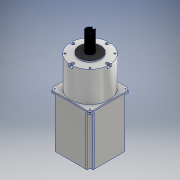
# Autodesk Inventor part: Nema 23 Stepper Motor
Saved by Autodesk Inventor 2018 (Build 220112000, 112)
## iProperties
Created: 2017-11-21
Part Number: Nema 23 Stepper Motor
Material: Generic
Document SubType Name: Modeling
Designer: p447144
Density: 1 g/cm^3
Appearance: Aluminum - Flat
Author: p447144
Autodesk Inventor part; units mm, degrees
ref_plane "YZ Plane" through (0, 0, 0) normal (1, 0, 0) x (0, 1, 0)
ref_plane "XY Plane" through (0, 0, 0) normal (0, 0, 1) x (1, 0, 0)
sketch "Sketch1" plane through (0, 0, 0) normal (0, 0, 1) x (1, 0, 0)
  line L0 (-28.5, -28.5) -> (28.5, -28.5)
  line L1 (28.5, -28.5) -> (28.5, 28.5)
  line L2 (28.5, 28.5) -> (-28.5, 28.5)
  line L3 (-28.5, 28.5) -> (-28.5, -28.5)
  arc A0 (23.5, 28.5) -> (28.5, 23.5) centre (28.5, 28.5) ccw
  line L4 (0, 28.5) -> (0, -28.5) construction
  line L5 (-28.5, 0) -> (28.5, 0) construction
  arc A1 (-28.5, 23.5) -> (-23.5, 28.5) centre (-28.5, 28.5) ccw
  arc A2 (28.5, -23.5) -> (23.5, -28.5) centre (28.5, -28.5) ccw
  arc A3 (-23.5, -28.5) -> (-28.5, -23.5) centre (-28.5, -28.5) ccw
  point P0 (0, 0)
  dimension "d0" = 57
  dimension "d1" = 57
  dimension "d2" = 10
  constraints: 12 end point, 8 point on circle, 8 point on line, 4 centre point, 4 midpoint, 3 symmetric about line, 2 parallel, 1 coincident, 1 horizontal, 1 perpendicular, 3 other
  measures "d0" distance of L2.end L1.end
  measures "d1" distance of L1.end L0.end
  measures "d2" diameter of A0
extrude "Extrusion1" add sketch "Sketch1" along normal blind 73 contours A3 L3 A1 L2 A0 L1 A2 L0
sketch "Sketch2" plane through (0, 0, 73) normal (0, 0, 1) x (1, 0, 0)
  line L0 (-28.5, -28.5) -> (28.5, -28.5)
  line L1 (28.5, -28.5) -> (28.5, 28.5)
  line L2 (28.5, 28.5) -> (-28.5, 28.5)
  line L3 (-28.5, 28.5) -> (-28.5, -28.5)
  line L4 (-28.5, -28.5) -> (28.5, 28.5) construction
  line L5 (28.5, -28.5) -> (-28.5, 28.5) construction
  point P0 (0, 0)
  dimension "d5" = 57
  dimension "d6" = 57
  constraints: 12 end point, 2 midpoint, 2 parallel, 1 horizontal, 1 perpendicular
  measures "d5" distance of L2.end L1.end
  measures "d6" distance of L1.end L0.end
extrude "Extrusion2" add sketch "Sketch2" along normal blind 3
sketch "Sketch3" plane through (0, 0, 76) normal (0, 0, 1) x (1, 0, 0)
  arc A0 (-28.5, 23.5) -> (-23.5, 28.5) centre (-28.5, 28.5) ccw projected
  line L0 (-28.5, 23.5) -> (-18.5, 23.5) construction
  line L1 (-23.5, 28.5) -> (-28.5, 28.5) projected
  line L2 (-23.5, 28.5) -> (-23.5, 18.5) construction
  line L3 (-23.5, 28.5) -> (-13.5, 28.5) construction
  line L4 (-28.5, 28.5) -> (-23.5, 23.5) construction
  line L5 (-23.5, 28.5) -> (-28.5, 23.5) construction
  circle A1 centre (-26, 26) radius 0.75
  line L6 (23.5, 28.5) -> (-23.5, 28.5) projected
  line L7 (0, 28.5) -> (0, -28.5) construction
  line L8 (-23.5, -28.5) -> (23.5, -28.5) projected
  line L9 (28.5, -23.5) -> (28.5, 23.5) projected
  line L10 (-28.5, 23.5) -> (-28.5, -23.5) projected
  line L11 (-28.5, 0) -> (28.5, 0) construction
  circle A2 centre (26, 26) radius 0.75
  line L12 (28.5, 0) -> (-28.5, 0) construction
  circle A3 centre (-26, -26) radius 0.75
  circle A4 centre (26, -26) radius 0.75
  point P0 (0, 0)
  dimension "d9" = 10
  dimension "d11" = 10
  dimension "d12" = 90
  dimension "d13" = 1.5
  constraints: 16 end point, 6 midpoint, 5 symmetric about line, 4 centre point, 2 horizontal, 1 perpendicular, 1 tangent, 1 vertical, 3 other
  measures "d9" distance of L0.start L0.end
  measures "d11" distance of L1.start L2.end
  measures "d12" angle of L2 L3
  measures "d13" diameter of A1
extrude "Extrusion3" cut sketch "Sketch3" against normal blind 3
sketch "Sketch4" plane through (0, 0, 76) normal (0, 0, 1) x (1, 0, 0)
  line L0 (-29.5, -29.5) -> (29.5, -29.5)
  line L1 (29.5, -29.5) -> (29.5, 29.5)
  line L2 (29.5, 29.5) -> (-29.5, 29.5)
  line L3 (-29.5, 29.5) -> (-29.5, -29.5)
  line L4 (29.5, -29.5) -> (-29.5, 29.5) construction
  line L5 (-29.5, 26) -> (-26, 29.5)
  line L6 (0, 29.5) -> (0, -29.5) construction
  line L7 (-29.5, 0) -> (29.5, 0) construction
  line L8 (29.5, 26) -> (26, 29.5)
  line L9 (-26, -29.5) -> (-29.5, -26)
  line L10 (26, -29.5) -> (29.5, -26)
  point P0 (0, 0)
  dimension "d16" = 59
  dimension "d17" = 59
  constraints: 22 end point, 8 point on line, 5 midpoint, 2 parallel, 2 perpendicular, 1 horizontal
  measures "d16" distance of L2.end L1.end
  measures "d17" distance of L1.end L0.end
extrude "Extrusion4" add sketch "Sketch4" along normal blind 2 contours L9 L3 L5 L2 L8 L1 L10 L0
sketch "Sketch5" plane through (0, 0, 78) normal (0, 0, 1) x (1, 0, 0)
  circle A0 centre (26, 26) radius 0.75 projected
  circle A1 centre (26, -26) radius 0.75 projected
  circle A2 centre (-26, -26) radius 0.75 projected
  circle A3 centre (-26, 26) radius 0.75 projected
  circle A4 centre (-26, 26) radius 0.75 projected
  circle A5 centre (-26, 26) radius 0.75
  circle A6 centre (26, 26) radius 0.75
  circle A7 centre (26, -26) radius 0.75
  circle A8 centre (-26, -26) radius 0.75
  point P0 (0, 0)
  constraints: 4 centre point, 4 coincident, 3 concentric
extrude "Extrusion5" cut sketch "Sketch5" against normal blind 2
sketch "Sketch6" plane through (0, 0, 78) normal (0, 0, 1) x (1, 0, 0)
  circle A0 centre (0, 0) radius 28.5
  constraints: 1 centre point, 1 coincident
extrude "Extrusion6" add sketch "Sketch6" along normal blind 45
sketch "Sketch7" plane through (0, 0, 123) normal (0, 0, 1) x (1, 0, 0)
  circle A0 centre (0, 0) radius 22.5 construction
  circle A1 centre (0, 0) radius 25 construction
  arc A2 (2, -25) -> (-2, -25) centre (0, -25) ccw
  circle A3 centre (0, 0) radius 28.5 projected
  line L0 (28.5, -27) -> (28.5, 27) projected
  line L1 (-28.5, 27) -> (-28.5, -27) projected
  line L2 (-23.5, -28.5) -> (23.5, -28.5) projected
  line L3 (-2, -23.5) -> (4, -23.5) construction
  line L4 (-2, -24.9199) -> (-2, -28.4297)
  line L5 (2, -24.9199) -> (2, -28.4297)
  arc A4 (-25, -2) -> (-25, 2) centre (-25, 0) ccw
  line L6 (-29.5, 26) -> (-29.5, -26) projected
  line L7 (-23, 2) -> (-15, 2) construction
  line L8 (-24.9199, 2) -> (-28.4297, 2)
  line L9 (-24.9199, -2) -> (-28.4297, -2)
  arc A5 (-2, 25) -> (2, 25) centre (0, 25) ccw
  line L10 (-2, 20.4297) -> (-2, 28.4297)
  line L11 (2, 20.4297) -> (2, 28.4297)
  line L12 (2, 20.4297) -> (10, 20.4297) construction
  line L13 (29.5, -26) -> (29.5, 26) projected
  arc A6 (25.08, 1.9984) -> (25.08, -1.9984) centre (25, 0) ccw
  line L14 (24.92, -1.9984) -> (28.4299, -1.9984)
  line L15 (24.92, 1.9984) -> (28.4299, 1.9984)
  circle A7 centre (-15, 16.7705) radius 1.5
  circle A8 centre (15, 16.7705) radius 1.5
  circle A9 centre (15, -16.7705) radius 1.5
  circle A10 centre (-15, -16.7705) radius 1.5
  circle A11 centre (-15, 16.7705) radius 1.5
  dimension "d26" = 50
  dimension "d25" = 45
  dimension "d28" = 4
  dimension "d32" = 4
  dimension "d39" = 4
  dimension "d40" = 8
  dimension "d41" = 8
  dimension "d42" = 90
  dimension "d46" = 4
  dimension "d83" = 3
  dimension "d84" = 3
  dimension "d85" = 3
  dimension "d86" = 3
  constraints: 22 end point, 14 point on circle, 10 centre point, 8 point on line, 5 horizontal, 4 vertical, 3 coincident, 1 concentric, 1 perpendicular, 22 other
  measures "d25" diameter of A0
  measures "d28" diameter of A2
  measures "d32" diameter of A4
  measures "d39" diameter of A5
  measures "d40" distance of L10.start L10.end
  measures "d41" distance of L11.start L11.end
  measures "d42" angle of L12 L11
  measures "d46" diameter of A6
  measures "d83" diameter of A7
  measures "d84" diameter of A8
  measures "d85" diameter of A9
  measures "d86" diameter of A10
extrude "Extrusion7" cut sketch "Sketch7" against normal blind 4 contours L5 A3 L4 A2 | L14 A6 L15 A3 | A3 L8 A4 L9 | L11 A5 L10 A3
fillet "Fillet1" radius 1 8 edges at (-2, -28.4297, 121) (2, -28.4297, 121) (28.4299, -1.9984, 121) (28.4299, 1.9984, 121) (-2, 28.4297, 121) (2, 28.4297, 121) (-28.4297, -2, 121) (-28.4297, 2, 121)
sketch "Sketch8" plane through (0, 0, 123) normal (0, 0, 1) x (1, 0, 0)
  circle A0 centre (0, 0) radius 16
  dimension "d52" = 32
  constraints: 1 centre point, 1 coincident
  measures "d52" diameter of A0
extrude "Extrusion8" add sketch "Sketch8" along normal blind 2
sketch "Sketch9" plane through (0, 0, 125) normal (0, 0, 1) x (1, 0, 0)
  circle A0 centre (0, 0) radius 6
  dimension "d55" = 12
  constraints: 1 centre point, 1 coincident
  measures "d55" diameter of A0
extrude "Extrusion9" add sketch "Sketch9" along normal blind 28
ref_plane "Work Plane1" through (0, 6, 0) normal (0, 1, 0) x (-1, 0, 0)
sketch "Sketch10" plane through (0, 6, 0) normal (0, 1, 0) x (-1, 0, 0)
  line L0 (6, 153) -> (-6, 153) projected
  line L1 (-6, 125) -> (6, 125) projected
  line L2 (6, 125) -> (6, 153) projected
  line L3 (-6, 125) -> (-6, 153) projected
  line L4 (6, 153) -> (-6, 153) projected
  line L5 (0, 153) -> (0, 143) construction
  line L6 (2, 133) -> (-2, 133)
  line L7 (-2, 133) -> (-2, 153)
  line L8 (-2, 153) -> (2, 153)
  line L9 (2, 153) -> (2, 133)
  line L10 (2, 133) -> (-2, 153) construction
  line L11 (-2, 133) -> (2, 153) construction
  line L12 (0, 133) -> (0, 135) construction
  arc A0 (-2, 135) -> (2, 135) centre (0, 135) ccw
  point P0 (0, 0)
  dimension "d66" = 10
  dimension "d67" = 4
  dimension "d68" = 2
  constraints: 16 end point, 4 midpoint, 3 point on circle, 3 point on line, 2 parallel, 2 vertical, 1 centre point, 1 coincident, 1 horizontal, 1 perpendicular
  measures "d66" distance of L5.start L5.end
  measures "d67" distance of L7.end L8.end
  measures "d68" distance of L12.start L12.end
extrude "Extrusion10" cut sketch "Sketch10" against normal blind 2.5 contours L9 A0 L7 L0
fillet "Fillet2" radius 1 8 edges at (-28.5, 23.5, 36.5) (-23.5, 28.5, 36.5) (23.5, 28.5, 36.5) (28.5, 23.5, 36.5) (23.5, -28.5, 36.5) (28.5, -23.5, 36.5) (-23.5, -28.5, 36.5) (-28.5, -23.5, 36.5)
fillet "Fillet3" radius 1 4 edges at (-28.5, 28.5, 74.5) (-28.5, -28.5, 74.5) (28.5, -28.5, 74.5) (28.5, 28.5, 74.5)
fillet "Fillet4" radius 1 16 edges at (23.2294, 28.2638, 0) (0, 28.5, 0) (-23.2294, 28.2638, 0) (-24.9645, 24.9645, 0) (-28.2638, 23.2294, 0) (-28.5, 0, 0) (-28.2638, -23.2294, 0) (-24.9645, -24.9645, 0) (-23.2294, -28.2638, 0) (0, -28.5, 0) (23.2294, -28.2638, 0) (24.9645, -24.9645, 0) (28.2638, -23.2294, 0) (28.5, 0, 0) (28.2638, 23.2294, 0) (24.9645, 24.9645, 0)
sketch "Sketch11" plane through (0, 0, 0) normal (0, 0, -1) x (-1, 0, 0)
  circle A0 centre (0, 0) radius 6 projected
  circle A1 centre (0, 0) radius 6
  constraints: 1 centre point, 1 coincident
extrude "Extrusion11" cut sketch "Sketch11" against normal blind 3
sketch "Sketch12" plane through (0, 0, 3) normal (0, 0, -1) x (-1, 0, 0)
  circle A0 centre (0, 0) radius 4
  dimension "d76" = 8
  constraints: 1 centre point, 1 coincident
  measures "d76" diameter of A0
extrude "Extrusion12" add sketch "Sketch12" along normal blind 2
sketch "Sketch13" plane through (0, 0, 1) normal (0, 0, -1) x (-1, 0, 0)
  circle A0 centre (0, 0) radius 4 projected
  circle A1 centre (0, 0) radius 0.5
  dimension "d79" = 1
  constraints: 1 centre point, 1 coincident
  measures "d79" diameter of A1
extrude "Extrusion13" cut sketch "Sketch13" against normal blind 2 contours A1
sketch "Sketch15" plane through (0, 0, 123) normal (0, 0, 1) x (1, 0, 0)
  circle A0 centre (0, 0) radius 6 projected
  circle A1 centre (0, 0) radius 26.0003 construction
  circle A2 centre (-26, 26) radius 0.75 construction
  circle A3 centre (0, 0) radius 0.5 construction
  line L0 (-26, 26) -> (0, 0) construction
  circle A4 centre (26, 26) radius 0.75 construction
  line L1 (0, 0) -> (26, 26) construction
  circle A5 centre (-26, -26) radius 0.75 construction
  line L2 (-26, -26) -> (0, 0) construction
  line L3 (26, -26) -> (0, 0) construction
  circle A6 centre (-18.385, 18.385) radius 1.5
  circle A7 centre (18.385, 18.385) radius 1.5
  circle A8 centre (-18.385, -18.385) radius 1.5
  circle A9 centre (18.385, -18.385) radius 1.5
  line L4 (18.385, -18.385) -> (-18.385, -18.385)
  dimension "d89" = 3
  dimension "d90" = 3
  dimension "d91" = 3
  dimension "d92" = 3
  dimension "d108" = 36.77
  constraints: 10 end point, 5 centre point, 4 point on circle, 4 point on line, 3 perpendicular, 1 coincident, 1 horizontal
  measures "d89" diameter of A6
  measures "d90" diameter of A7
  measures "d91" diameter of A8
  measures "d92" diameter of A9
  measures "d108" distance of L4.start L4.end
hole "Hole1" at (-18.385, 18.385, 123) at (18.385, 18.385, 123) at (-18.385, -18.385, 123) at (18.385, -18.385, 123) direction (0, 0, -1) diameter 2.487 depth 9.525 tip angle 118 thread size "5-40 UNC" class "2B" standard "ANSI Unified Screw Threads"
thread "Thread1" size "M1.6x0.35" class "6H" standard "ANSI Metric M Profile" full length
thread "Thread2" size "M1.6x0.35" class "6H" standard "ANSI Metric M Profile" full length
thread "Thread3" size "M1.6x0.35" class "6H" standard "ANSI Metric M Profile" full length
thread "Thread4" size "M1.6x0.35" class "6H" standard "ANSI Metric M Profile" full length
body "Solid1"
